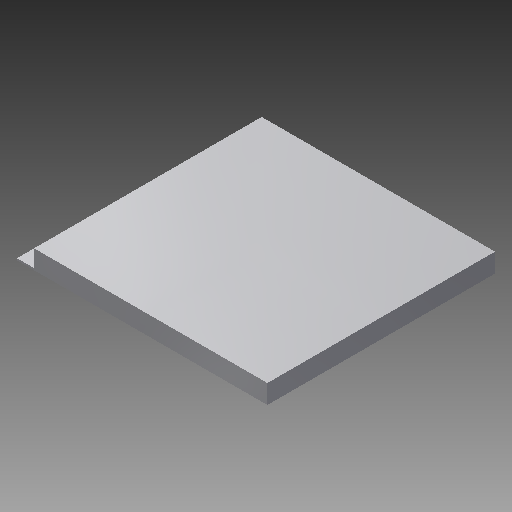
# Autodesk Inventor part: peltier
Saved by Autodesk Inventor 2019.2 (Build 232265000, 265)
## iProperties
Created: 2007-07-04
Part Number: peltier
Document SubType Name: Modeling
Designer: Administrator
Density: 1 g/cm^3
Material: Generic
Appearance: Smooth - White
Author: Administrator
Autodesk Inventor part; units mm, degrees
ref_plane "YZ Plane" through (0, 0, 0) normal (1, 0, 0) x (0, 1, 0)
ref_plane "XZ Plane" through (0, 0, 0) normal (0, 1, 0) x (-1, 0, 0)
ref_plane "XY Plane" through (0, 0, 0) normal (0, 0, 1) x (1, 0, 0)
sketch "Sketch1" plane through (0, 0, 0) normal (0, 0, 1) x (1, 0, 0)
  line L0 (-24.8062, 29.3057) -> (19.0938, 29.3057)
  line L1 (19.0938, 29.3057) -> (19.0938, -10.5943)
  line L2 (19.0938, -10.5943) -> (-24.8062, -10.5943)
  line L3 (-24.8062, -10.5943) -> (-24.8062, 29.3057)
  dimension "d0" = 39.9
  dimension "d1" = 43.9
  constraints: 8 end point, 2 parallel, 1 horizontal, 1 perpendicular
  measures "d0" distance between parallel lines of L2 L0
  measures "d1" distance between parallel lines of L1 L3
extrude "Extrusion1" add sketch "Sketch1" along normal blind 3.33
sketch "Sketch2" plane through (0, 0, 3.33) normal (0, 0, 1) x (1, 0, 0)
  line L0 (19.0938, -10.5943) -> (-24.8062, -10.5943) projected
  line L1 (-24.8062, 29.3057) -> (-21.8062, 29.3057)
  line L2 (-21.8062, 29.3057) -> (-21.8062, -10.5943)
  line L3 (-21.8062, -10.5943) -> (-24.8062, -10.5943)
  line L4 (-24.8062, -10.5943) -> (-24.8062, 29.3057)
  dimension "d4" = 3
  constraints: 8 end point, 2 parallel, 1 horizontal, 1 perpendicular, 1 point on line
  measures "d4" distance between parallel lines of L2 L4
extrude "Extrusion2" cut sketch "Sketch2" against normal blind 3
sketch "Sketch3" plane through (-24.8062, -10.5943, 0) normal (0, -1, 0) x (1, 0, 0)
  line L0 (3, 3.33) -> (3, 0.33) projected
  line L1 (3, 0.33) -> (0, 0.33) projected
  line L2 (0, 0) -> (0, 0.33) projected
  line L3 (43.9, 0) -> (0, 0) projected
  line L4 (43.9, 0) -> (43.9, 3.33) projected
  line L5 (43.9, 3.33) -> (3, 3.33) projected
  dimension "d7" = 3.33
  measures "d7" distance between parallel lines of L3 L5
body "Solid1"
